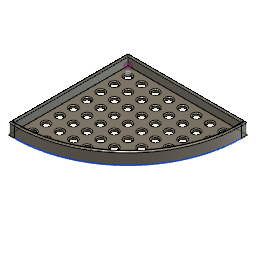
Bathroom_Shelf (Autodesk Fusion 360 design; units mm, degrees)
Autodesk Fusion 360 part; units mm, degrees
note: some values were not read from the file. Chosen so that the rebuilt part matches the saved one: which face or edge a step refers to. Set by a fixed rule: which sketch regions a step uses.
sketch "Sketch1" plane through (0, 0, 0) normal (0, 1, 0) x (1, 0, 0)
  line L0 (0, 0) -> (200, 0)
  line L1 (200, 0) -> (200, -10)
  line L2 (10, -200) -> (0, -200)
  line L3 (0, -200) -> (0, 0)
  arc A0 (10, -200) -> (200, -10) centre (10, -10) ccw
  dimension "d1" = 200
  dimension "d2" = 200
extrude "Extrude1" add sketch "Sketch1" along normal blind 20
shell "Shell1" thickness 5 removed faces 1 at (96.0053, 20, 96.0053)
fillet "Fillet1" radius 2 3 edges at (5, 20, 200) (144.3503, 20, 144.3503) (200, 20, 5)
fillet "Fillet2" radius 2 11 edges at (200, 9, 0) (199.4142, 19.4142, 0) (99, 20, 0) (0, 20, 99) (7.5, 20, 195) (5, 20, 100) (100, 20, 5) (195, 20, 7.5) (140.8148, 20, 140.8148) (0, 9, 200) (0, 19.4142, 199.4142)
sketch "Sketch2" plane through (0, 5, 0) normal (0, 1, 0) x (-1, 0, 0)
  arc A0 (-10, 195) -> (-195, 10) centre (-10, 10) ccw
  line L0 (-195, 5) -> (-5, 5)
  line L1 (-5, 5) -> (-5, 195)
  circle A1 centre (-20, 20) radius 5
  circle A2 centre (-42.8571, 20) radius 5
  circle A3 centre (-65.7143, 20) radius 5
  circle A4 centre (-88.5714, 20) radius 5
  circle A5 centre (-111.4286, 20) radius 5
  circle A6 centre (-134.2857, 20) radius 5
  circle A7 centre (-157.1429, 20) radius 5
  circle A8 centre (-180, 20) radius 5
  circle A9 centre (-65.7143, 42.8571) radius 5
  circle A10 centre (-111.4286, 42.8571) radius 5
  circle A11 centre (-134.2857, 42.8571) radius 5
  circle A12 centre (-157.1429, 42.8571) radius 5
  circle A13 centre (-20, 42.8571) radius 5
  circle A14 centre (-88.5714, 42.8571) radius 5
  circle A15 centre (-42.8571, 42.8571) radius 5
  circle A16 centre (-180, 42.8571) radius 5
  circle A17 centre (-65.7143, 65.7143) radius 5
  circle A18 centre (-111.4286, 65.7143) radius 5
  circle A19 centre (-134.2857, 65.7143) radius 5
  circle A20 centre (-157.1429, 65.7143) radius 5
  circle A21 centre (-20, 65.7143) radius 5
  circle A22 centre (-88.5714, 65.7143) radius 5
  circle A23 centre (-42.8571, 65.7143) radius 5
  circle A24 centre (-65.7143, 88.5714) radius 5
  circle A25 centre (-111.4286, 88.5714) radius 5
  circle A26 centre (-134.2857, 88.5714) radius 5
  circle A27 centre (-157.1429, 88.5714) radius 5
  circle A28 centre (-20, 88.5714) radius 5
  circle A29 centre (-88.5714, 88.5714) radius 5
  circle A30 centre (-42.8571, 88.5714) radius 5
  circle A31 centre (-65.7143, 111.4286) radius 5
  circle A32 centre (-111.4286, 111.4286) radius 5
  circle A33 centre (-134.2857, 111.4286) radius 5
  circle A34 centre (-20, 111.4286) radius 5
  circle A35 centre (-88.5714, 111.4286) radius 5
  circle A36 centre (-42.8571, 111.4286) radius 5
  circle A37 centre (-65.7143, 134.2857) radius 5
  circle A38 centre (-111.4286, 134.2857) radius 5
  circle A39 centre (-20, 134.2857) radius 5
  circle A40 centre (-88.5714, 134.2857) radius 5
  circle A41 centre (-42.8571, 134.2857) radius 5
  circle A42 centre (-65.7143, 157.1429) radius 5
  circle A43 centre (-20, 157.1429) radius 5
  circle A44 centre (-88.5714, 157.1429) radius 5
  circle A45 centre (-42.8571, 157.1429) radius 5
  circle A46 centre (-20, 180) radius 5
  circle A47 centre (-42.8571, 180) radius 5
  line L2 (-5, 195) -> (-10, 195)
  line L3 (-195, 10) -> (-195, 5)
  dimension "d9" = 10
  dimension "d15" = -160
  dimension "d16" = 0
  dimension "d19" = 0
  dimension "d20" = 160
  measures "d9" diameter of A1
extrude "Extrude4" cut sketch "Sketch2" against normal blind 15 contours A1 | A2 | A3 | A4 | A5 | A6 | A7 | A8 | A9 | A10 | A11 | A12 | A13 | A14 | A15 | A16 | A17 | A18 | A19 | A20 | A21 | A22 | A23 | A24 | A25 | A26 | A27 | A28 | A29 | A30 | A31 | A32 | A33 | A34 | A35 | A36 | A37 | A38 | A39 | A40 | A41 | A42 | A43 | A44 | A45 | A46 | A47
fillet "Fillet5" radius 2 94 edges at (25, 0, 180) (47.8571, 0, 180) (25, 0, 157.1429) (47.8571, 0, 157.1429) (70.7143, 0, 157.1429) (93.5714, 0, 157.1429) (25, 0, 134.2857) (47.8571, 0, 134.2857) (25, 0, 111.4286) (47.8571, 0, 111.4286) (70.7143, 0, 134.2857) (93.5714, 0, 134.2857) (70.7143, 0, 111.4286) (93.5714, 0, 111.4286) (116.4286, 0, 134.2857) (116.4286, 0, 111.4286) (139.2857, 0, 111.4286) (25, 0, 88.5714) (47.8571, 0, 88.5714) (25, 0, 65.7143) (47.8571, 0, 65.7143) (70.7143, 0, 88.5714) (93.5714, 0, 88.5714) (70.7143, 0, 65.7143) (93.5714, 0, 65.7143) (25, 0, 42.8571) (47.8571, 0, 42.8571) (25, 0, 20) (47.8571, 0, 20) (70.7143, 0, 42.8571) (93.5714, 0, 42.8571) (70.7143, 0, 20) (93.5714, 0, 20) (116.4286, 0, 88.5714) (139.2857, 0, 88.5714) (116.4286, 0, 65.7143) (139.2857, 0, 65.7143) (162.1429, 0, 88.5714) (162.1429, 0, 65.7143) (116.4286, 0, 42.8571) (139.2857, 0, 42.8571) (116.4286, 0, 20) (139.2857, 0, 20) (162.1429, 0, 42.8571) (185, 0, 42.8571) (162.1429, 0, 20) (185, 0, 20) (25, 5, 180) (47.8571, 5, 180) (25, 5, 157.1429) (47.8571, 5, 157.1429) (70.7143, 5, 157.1429) (93.5714, 5, 157.1429) (25, 5, 134.2857) (47.8571, 5, 134.2857) (25, 5, 111.4286) (47.8571, 5, 111.4286) (70.7143, 5, 134.2857) (93.5714, 5, 134.2857) (70.7143, 5, 111.4286) (93.5714, 5, 111.4286) (116.4286, 5, 134.2857) (116.4286, 5, 111.4286) (139.2857, 5, 111.4286) (25, 5, 88.5714) (47.8571, 5, 88.5714) (25, 5, 65.7143) (47.8571, 5, 65.7143) (70.7143, 5, 88.5714) (93.5714, 5, 88.5714) (70.7143, 5, 65.7143) (93.5714, 5, 65.7143) (25, 5, 42.8571) (47.8571, 5, 42.8571) (25, 5, 20) (47.8571, 5, 20) (70.7143, 5, 42.8571) (93.5714, 5, 42.8571) (70.7143, 5, 20) (93.5714, 5, 20) (116.4286, 5, 88.5714) (139.2857, 5, 88.5714) (116.4286, 5, 65.7143) (139.2857, 5, 65.7143) (162.1429, 5, 88.5714) (162.1429, 5, 65.7143) (116.4286, 5, 42.8571) (139.2857, 5, 42.8571) (116.4286, 5, 20) (139.2857, 5, 20) (162.1429, 5, 42.8571) (185, 5, 42.8571) (162.1429, 5, 20) (185, 5, 20)
extrude "Extrude3" cut sketch "Sketch2" against normal blind 15 draft 10 contours A1 | A2 | A3 | A4 | A5 | A6 | A7 | A8 | A9 | A10 | A11 | A12 | A13 | A14 | A15 | A16 | A17 | A18 | A19 | A20 | A21 | A22 | A23 | A24 | A25 | A26 | A27 | A28 | A29 | A30 | A31 | A32 | A33 | A34 | A35 | A36 | A37 | A38 | A39 | A40 | A41 | A42 | A43 | A44 | A45 | A46 | A47
fillet "Fillet4" [no effect]
extrude "Extrude2" cut sketch "Sketch2" against normal blind 15 contours A1
fillet "Fillet3" [no effect]
sketch "Sketch3" plane through (0, 0, 0) normal (1, 0, 0) x (0, 0, -1)
named bodies: "Shelf"
